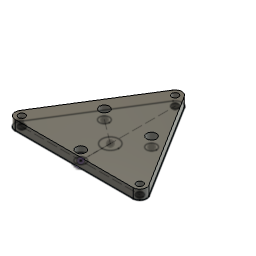
_TheFlag.7fe9db87-e2a5-4b7a-a887-d6b63744287c (Autodesk Fusion 360 design; units mm, degrees)
Autodesk Fusion 360 part; units mm, degrees
sketch "Sketch1" plane through (0, 0, 0) normal (0, 1, 0) x (1, 0, 0)
  circle A0 centre (0, 40) radius 1.4
  circle A1 centre (-25, 0) radius 1.4
  circle A2 centre (25, 0) radius 1.4
  line L0 (-25, 0) -> (25, 0) construction
  line L1 (0, 0) -> (0, 40) construction
  line L2 (-27.3744, 1.484) -> (-2.3744, 41.484)
  line L3 (25, -2.8) -> (-25, -2.8)
  line L4 (27.3744, 1.484) -> (2.3744, 41.484)
  arc A3 (25, -2.8) -> (27.3744, 1.484) centre (25, 0) ccw
  arc A4 (-27.3744, 1.484) -> (-25, -2.8) centre (-25, 0) ccw
  arc A5 (2.3744, 41.484) -> (-2.3744, 41.484) centre (0, 40) ccw
  circle A6 centre (-10, 20) radius 2.05
  circle A7 centre (10, 20) radius 2.05
  circle A8 centre (0, 0) radius 2.05
  line L5 (0, 0) -> (0, -2.8) construction
  circle A9 centre (0, 12.5) radius 3.5
  line L6 (0, 12.5) -> (-10, 20) construction
  line L7 (0, 12.5) -> (0, 0) construction
  dimension "d16" = 2.8
  dimension "d19" = 50
  dimension "d21" = 40
  dimension "d22" = 1.4
  dimension "d23" = 1.4
  dimension "d24" = 4.1
  dimension "d28" = 7
  dimension "d36" = 20
  dimension "d37" = 10
  constraint coincident A1.centre L0.start
  constraint coincident A2.centre L0.end
  constraint horizontal L0
  constraint midpoint L0 L1.start
  constraint coincident A0.centre L1.end
  constraint vertical L1
  constraint equal A0 A2
  constraint equal A1 A2
  constraint parallel L0 L3
  constraint symmetric L1 L2.start L4.start
  constraint symmetric L1 L2.end L4.end
  constraint tangent L3 A3
  constraint tangent L4 A3
  constraint symmetric L1 L3.start L3.end
  constraint symmetric L1 L4.start L2.start
  constraint symmetric L1 A3 A4
  constraint coincident L2 A4.start
  constraint tangent L2 A4
  constraint tangent L4 A5
  constraint coincident L4.start A3.end
  constraint symmetric L1 A6 A7
  constraint coincident L1.start A8.centre
  constraint equal A7 A8
  constraint midpoint L3 L5.end
  constraint coincident L1 A9.centre
  constraint coincident A9.centre L6.start
  constraint coincident A6.centre L6.end
  constraint perpendicular L0 L7
  constraint equal L6 L7
  measures "d16" diameter of A0
  measures "d19" horizontal distance of A1.centre A2.centre
  measures "d21" distance of L1.start A0.centre
  measures "d22" distance of A0 A5
  measures "d23" distance of A2 A3
  measures "d24" diameter of A7
  measures "d28" diameter of A9
  measures "d36" vertical distance of A7.centre L1.start
  measures "d37" horizontal distance of A7.centre L1.start
extrude "Extrude1" add sketch "Sketch1" along normal blind 4 contours L2 L3 L4 A3 A4 A5 | A9 makes body 1
extrude "Extrude2" add sketch "Sketch1" along normal blind 7.5 separate body contours A0 | A1 | A2 | L2 L3 L4 A3 A4 A5 makes body 2
extrude "Extrude3" add sketch "Sketch1" along normal blind 1 contours A0 | A1 | A2 bodies 1
extrude "Extrude5" add sketch "Sketch1" along normal blind 1 contours A6 | A7 | A8 bodies 2
extrude "Extrude6" add sketch "Sketch1" along normal blind 5 separate body contours L2 L3 L4 A3 A4 A5 | A6 | A7 | A8 | A9 makes body 3
hidden bodies 2 3
equation "holeDiam = 2.8 mm"
equation "RodHoleDiam = 4.1 mm"
equation "d16 = holeDiam"
equation "d22 = holeDiam / 2"
equation "d23 = holeDiam / 2"
equation "d24 = RodHoleDiam"
named bodies: "Flagpbot", "Flagtop", "Strengtheners"
